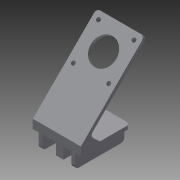
# Autodesk Inventor part: slider
Saved by Autodesk Inventor 2015 (Build 190159000, 159)
## iProperties
Created: 2014-11-15
Part Number: slider
Material: Generic
Document SubType Name: Modeling
Designer: Rene
Density: 1 g/cm^3
Appearance: Default
Author: Rene
Autodesk Inventor part; units mm, degrees
ref_plane "YZ Plane" through (0, 0, 0) normal (1, 0, 0) x (0, 1, 0)
ref_plane "XZ Plane" through (0, 0, 0) normal (0, 1, 0) x (-1, 0, 0)
ref_plane "XY Plane" through (0, 0, 0) normal (0, 0, 1) x (1, 0, 0)
sketch "Sketch1" plane through (0, 0, 0) normal (0, 1, 0) x (-1, 0, 0)
  line L0 (9.3294, -16.9333) -> (-32.5806, -16.9333)
  line L1 (-32.5806, -16.9333) -> (-32.5806, 33.8667)
  line L2 (-32.5806, 33.8667) -> (9.3294, 33.8667)
  line L3 (9.3294, 33.8667) -> (9.3294, -16.9333)
  point P0 (0, 0)
  dimension "d0" = 50.8
  dimension "d1" = 41.91
  constraints: 8 end point, 2 parallel, 1 horizontal, 1 perpendicular
  measures "d0" distance of L0.end L1.end
  measures "d1" distance of L1.end L2.end
extrude "Extrusion1" add sketch "Sketch1" along normal blind 3.175
chamfer "Chamfer1" distance 3.175 angle 45 1 edges at (11.6256, 3.175, 33.8667)
sketch "Sketch9" plane through (32.5806, 0, -16.9333) normal (1, 0, 0) x (0, 0, -1)
  line L0 (-47.625, 3.175) -> (0, 3.175) projected
  line L1 (-11.631, 34.6788) -> (-43.1349, 3.175) projected
  line L2 (-13.8761, 36.9239) -> (-11.631, 34.6788) projected
  line L3 (-34.9797, 11.3302) -> (-26.8245, 3.175)
  point P0 (-16.9333, 0)
  dimension "d15" = 33.02
  constraints: 2 end point, 2 point on line, 1 parallel
  measures "d15" distance between parallel lines of L2 L3
extrude "Extrusion4" add sketch "Sketch9" against normal blind 3.175
sketch "Sketch10" plane through (-9.3294, 0, -16.9333) normal (-1, 0, 0) x (0, 0, 1)
  line L0 (0, 3.175) -> (47.625, 3.175) projected
  line L1 (13.8761, 36.9239) -> (11.631, 34.6788) projected
  line L2 (43.1349, 3.175) -> (11.631, 34.6788) projected
  line L3 (34.9797, 11.3302) -> (26.8245, 3.175)
  point P0 (16.9333, 0)
  dimension "d18" = 33.02
  constraints: 2 end point, 2 point on line, 1 perpendicular
  measures "d18" distance between parallel lines of L1 L3
extrude "Extrusion5" add sketch "Sketch10" against normal blind 3.175
fillet "Fillet3" radius 3.175 2 edges at (-7.7419, 3.175, 9.8912) (30.9931, 3.175, 9.8912)
fillet "Fillet4" radius 3.175 2 edges at (-9.3294, 1.5875, -16.9333) (32.5806, 1.5875, -16.9333)
sketch "Sketch11" plane through (0, 0, 0) normal (0, -1, 0) x (1, 0, 0)
  line L0 (-9.3294, 26.2015) -> (32.5806, 26.2015) projected
  line L1 (-9.3294, 33.8667) -> (-9.3294, -13.7583) projected
  line L2 (-6.1544, -16.9333) -> (29.4056, -16.9333) projected
  line L3 (32.5806, -13.7583) -> (32.5806, 33.8667) projected
  line L4 (11.6256, 26.2015) -> (11.6256, -16.9333)
  line L5 (-9.3294, 0.8015) -> (32.5806, 0.8015)
  circle A0 centre (11.6256, 0.8015) radius 3.175
  point P0 (0, 0)
  dimension "d24" = 20.955
  dimension "d25" = 25.4
  dimension "d26" = 6.35
  constraints: 4 end point, 3 midpoint, 2 point on line, 1 centre point, 1 perpendicular
  measures "d24" distance between parallel lines of L1 L4
  measures "d25" distance between parallel lines of L0 L5
  measures "d26" diameter of A0
extrude "Extrusion9" cut sketch "Sketch11" against normal blind 12.446 contours A0 L5 L4 | L4 L5 A0 | L5 L4 A0 | L5 A0 L4
sketch "Sketch19" plane through (0, 0, 0) normal (0, -1, 0) x (1, 0, 0)
  circle A0 centre (11.6256, 0.8015) radius 3.175 projected
  circle A1 centre (11.6256, -9.3585) radius 3.175
  point P0 (0, 0)
  dimension "d44" = 6.35
  dimension "d45" = 10.16
  dimension "d46" = 0
  constraints: 1 centre point
  measures "d44" diameter of A1
  measures "d45" distance of A0.centre A1.centre
  measures "d46" horizontal distance of A0.centre A1.centre
extrude "Extrusion10" add sketch "Sketch19" along normal blind 12.446 contours A1
sketch "Sketch20" plane through (0, 0, 0) normal (0, -1, 0) x (1, 0, 0)
  circle A0 centre (11.6256, 0.8015) radius 3.175 projected
  circle A1 centre (11.6256, 10.9615) radius 3.175
  point P0 (0, 0)
  dimension "d49" = 6.35
  dimension "d50" = 10.16
  dimension "d51" = 0
  constraints: 1 centre point
  measures "d49" diameter of A1
  measures "d50" distance of A0.centre A1.centre
  measures "d51" horizontal distance of A0.centre A1.centre
extrude "Extrusion11" add sketch "Sketch20" along normal blind 12.446 contours A1
sketch "Sketch24" plane through (0, 0, 0) normal (0, -1, 0) x (1, 0, 0)
  circle A0 centre (11.6256, 0.8015) radius 3.175 projected
  line L0 (-9.3294, 26.2015) -> (32.5806, 26.2015) projected
  line L1 (-6.1544, -16.9333) -> (29.4056, -16.9333) projected
  line L2 (24.3256, 26.2015) -> (24.3256, -16.9333)
  line L3 (24.3256, 26.2015) -> (27.5006, 26.2015)
  line L4 (27.5006, 26.2015) -> (27.5006, -16.9333)
  line L5 (27.5006, -16.9333) -> (24.3256, -16.9333)
  line L6 (24.3256, -16.9333) -> (24.3256, 26.2015)
  point P0 (0, 0)
  dimension "d64" = 12.7
  dimension "d65" = 3.175
  constraints: 10 end point, 3 point on line, 2 parallel, 2 perpendicular, 1 horizontal
  measures "d64" distance from line of L2 A0.centre
  measures "d65" distance of L2.start L3.end
extrude "Extrusion14" add sketch "Sketch24" along normal blind 12.446 contours L0 L4 L1 L2
sketch "Sketch25" plane through (0, 0, 0) normal (0, -1, 0) x (1, 0, 0)
  circle A0 centre (11.6256, 0.8015) radius 3.175 projected
  line L0 (-9.3294, 26.2015) -> (24.3256, 26.2015) projected
  line L1 (-6.1544, -16.9333) -> (24.3256, -16.9333) projected
  line L2 (-1.0744, 26.2015) -> (-1.0744, -16.9333)
  line L3 (-1.0744, -16.9333) -> (-4.2494, -16.9333)
  line L4 (-4.2494, -16.9333) -> (-4.2494, 26.2015)
  line L5 (-4.2494, 26.2015) -> (-1.0744, 26.2015)
  line L6 (-1.0744, 26.2015) -> (-1.0744, -16.9333)
  point P0 (0, 0)
  dimension "d68" = 12.7
  dimension "d69" = 3.175
  constraints: 10 end point, 3 point on line, 2 parallel, 2 perpendicular, 1 horizontal
  measures "d68" distance from line of L2 A0.centre
  measures "d69" distance between parallel lines of L6 L4
extrude "Extrusion15" add sketch "Sketch25" along normal blind 12.446 contours L0 L2 L1 L4
fillet "Fillet8" radius 3.175 4 edges at (25.9131, -12.446, 26.2015) (25.9131, -12.446, -16.9333) (-2.6619, -12.446, -16.9333) (-2.6619, -12.446, 26.2015)
sketch "Sketch28" plane through (-9.3294, 3.175, 30.6917) normal (0, 0.7071068, 0.7071068) x (1, 0, 0)
  line L0 (41.91, -4.4901) -> (41.91, 0) projected
  line L1 (41.91, 0) -> (0, 0) projected
  line L2 (0, 0) -> (0, -4.4901) projected
  line L3 (41.91, -4.4901) -> (0, -4.4901) projected
  line L4 (0, -4.4901) -> (41.91, -4.4901)
  line L5 (41.91, -4.4901) -> (41.91, 85.0449)
  line L6 (41.91, 85.0449) -> (0, 85.0449)
  line L7 (0, 85.0449) -> (0, -4.4901)
  point P0 (9.3294, 19.4572)
  dimension "d75" = 41.91
  dimension "d76" = 89.535
  constraints: 8 end point, 2 parallel, 1 horizontal, 1 perpendicular
  measures "d75" distance between parallel lines of L5 L7
  measures "d76" distance between parallel lines of L3 L6
extrude "Extrusion16" add sketch "Sketch28" against normal blind 3.175 contours L1 L7 L6 L5
sketch "Sketch29" plane through (-9.3294, 0, 33.8667) normal (0, 0.7071068, 0.7071068) x (1, 0, 0)
  line L0 (41.91, 89.535) -> (0, 89.535) projected
  line L1 (0, 89.535) -> (0, 0) projected
  circle A0 centre (20.955, 68.58) radius 11.1125
  point P0 (9.3294, 23.9473)
  dimension "d79" = 22.225
  dimension "d80" = 20.955
  dimension "d81" = 20.955
  constraints: 1 centre point
  measures "d79" diameter of A0
  measures "d80" distance from line of L1 A0.centre
  measures "d81" distance from line of L0 A0.centre
extrude "Extrusion17" cut sketch "Sketch29" against normal blind 3.175
sketch "Sketch30" plane through (-9.3294, 0, 33.8667) normal (0, 0.7071068, 0.7071068) x (1, 0, 0)
  circle A0 centre (20.955, 68.58) radius 11.1125 projected
  circle A1 centre (5.461, 84.074) radius 1.7272
  point P0 (9.3294, 23.9473)
  dimension "d84" = 3.4544
  dimension "d85" = 15.494
  dimension "d86" = 15.494
  constraints: 1 centre point
  measures "d84" diameter of A1
  measures "d85" horizontal distance of A0.centre A1.centre
  measures "d86" horizontal distance of A0.centre A1.centre
extrude "Extrusion18" cut sketch "Sketch30" against normal blind 3.175 contours A1
sketch "Sketch31" plane through (-9.3294, 0, 33.8667) normal (0, 0.7071068, 0.7071068) x (1, 0, 0)
  circle A0 centre (5.461, 84.074) radius 1.7272 projected
  circle A1 centre (20.955, 68.58) radius 11.1125 projected
  circle A2 centre (5.461, 53.086) radius 1.7272
  point P0 (9.3294, 23.9473)
  dimension "d89" = 3.4544
  dimension "d90" = 3.4544
  dimension "d91" = 15.494
  dimension "d92" = 15.494
  constraints: 1 centre point
  measures "d89" diameter of A0
  measures "d90" diameter of A2
  measures "d91" horizontal distance of A1.centre A2.centre
  measures "d92" horizontal distance of A1.centre A2.centre
extrude "Extrusion19" cut sketch "Sketch31" against normal blind 3.175 contours A2
sketch "Sketch32" plane through (-9.3294, 0, 33.8667) normal (0, 0.7071068, 0.7071068) x (1, 0, 0)
  circle A0 centre (20.955, 68.58) radius 11.1125 projected
  circle A1 centre (36.449, 84.074) radius 1.7272
  point P0 (9.3294, 23.9473)
  dimension "d95" = 3.4544
  dimension "d96" = 15.494
  dimension "d97" = 15.494
  constraints: 1 centre point
  measures "d95" diameter of A1
  measures "d96" horizontal distance of A1.centre A0.centre
  measures "d97" horizontal distance of A0.centre A1.centre
extrude "Extrusion20" cut sketch "Sketch32" against normal blind 3.175 contours A1
sketch "Sketch33" plane through (-9.3294, 0, 33.8667) normal (0, 0.7071068, 0.7071068) x (1, 0, 0)
  circle A0 centre (20.955, 68.58) radius 11.1125 projected
  circle A1 centre (36.449, 53.086) radius 1.7272
  point P0 (9.3294, 23.9473)
  dimension "d100" = 3.4544
  dimension "d101" = 15.494
  dimension "d102" = 15.494
  constraints: 1 centre point
  measures "d100" diameter of A1
  measures "d101" horizontal distance of A1.centre A0.centre
  measures "d102" horizontal distance of A0.centre A1.centre
extrude "Extrusion21" cut sketch "Sketch33" against normal blind 3.175 contours A1
fillet "Fillet9" radius 3.175 2 edges at (-9.3294, 62.1883, -30.5667) (32.5806, 62.1883, -30.5667)
fillet "Fillet10" radius 3.175 2 edges at (30.9931, 11.3302, 18.0464) (-7.7419, 11.3302, 18.0464)
sketch "Sketch37" plane through (11.6256, -12.446, 10.9615) normal (0, -1, 0) x (1, 0, 0)
  line L0 (-15.875, 12.065) -> (-15.875, -24.7199) projected
  line L1 (-12.7, -24.7199) -> (-12.7, 12.065) projected
  circle A0 centre (0, 0) radius 3.175 projected
  line L2 (-3.175, 0) -> (3.175, 0)
  line L3 (3.175, 0) -> (3.175, 12.7)
  line L4 (3.175, 12.7) -> (-3.175, 12.7)
  line L5 (-3.175, 12.7) -> (-3.175, 0)
  point P0 (-11.6256, -10.9615)
  dimension "d111" = 3.175
  dimension "d112" = 6.35
  dimension "d113" = 12.7
  constraints: 8 end point, 2 parallel, 1 horizontal, 1 horizontal alignment, 1 perpendicular, 1 other
  measures "d111" distance between parallel lines of L0 L1
  measures "d112" distance between parallel lines of L5 L3
  measures "d113" distance of L4.end L2.start
extrude "Extrusion22" add sketch "Sketch37" against normal blind 12.954 contours L2 A0 | A0 L5 L4 L3 picked at (0.7922, 0.7018)
sketch "Sketch38" plane through (0, -12.446, 0) normal (0, -1, 0) x (1, 0, 0)
  line L0 (14.8006, 10.9615) -> (14.8006, 23.6615) projected
  line L1 (14.8006, 16.2386) -> (8.4506, 16.2386)
  line L2 (8.4506, 16.2386) -> (8.4506, 7.2793)
  line L3 (8.4506, 7.2793) -> (14.8006, 7.2793)
  line L4 (14.8006, 7.2793) -> (14.8006, 16.2386)
  point P0 (0, 0)
  dimension "d116" = 6.35
  constraints: 8 end point, 2 parallel, 1 horizontal, 1 perpendicular, 1 point on line
  measures "d116" distance between parallel lines of L2 L0
extrude "Extrusion23" add sketch "Sketch38" against normal blind 12.954
sketch "Sketch39" plane through (11.6256, -12.446, -9.3585) normal (0, -1, 0) x (1, 0, 0)
  line L0 (3.175, -3.175) -> (-3.175, -3.175)
  line L1 (-3.175, -3.175) -> (-3.175, 3.175)
  line L2 (-3.175, 3.175) -> (3.175, 3.175)
  line L3 (3.175, 3.175) -> (3.175, -3.175)
  point P0 (-11.6256, 9.3585)
  dimension "d119" = 6.35
  dimension "d120" = 6.35
  constraints: 8 end point, 2 parallel, 1 horizontal, 1 perpendicular
  measures "d119" distance of L0.end L1.end
  measures "d120" distance between parallel lines of L1 L3
extrude "Extrusion24" add sketch "Sketch39" against normal blind 12.954
fillet "Fillet12" radius 3.175 1 edges at (14.8006, -6.223, -12.5335)
fillet "Fillet13" radius 3.175 1 edges at (8.4506, -6.223, -12.5335)
sketch "Sketch44" plane through (32.5806, 0, 33.8667) normal (1, 0, 0) x (0, 0, -1)
  line L0 (7.6651, 0) -> (7.6651, 7.6651)
  line L1 (61.0657, 61.0657) -> (0, 0) projected
  line L2 (0, 0) -> (7.6651, 0)
  line L3 (47.625, 0) -> (0, 0) projected
  line L4 (7.6651, 7.6651) -> (0, 0)
  point P0 (33.8667, 0)
  constraints: 6 end point, 2 collinear, 1 point on line, 1 vertical
extrude "Extrusion25" cut sketch "Sketch44" against normal blind 76.2
sketch "Sketch45" plane through (-9.3294, 0.9299, 28.4466) normal (0, -0.7071068, -0.7071068) x (-1, 0, 0)
  line L0 (-38.735, 3.175) -> (-3.175, 3.175)
  line L1 (-3.175, 3.175) -> (-3.175, 34.1687)
  line L2 (-3.175, 34.1687) -> (-38.735, 34.1687)
  line L3 (-38.735, 34.1687) -> (-38.735, 3.175)
  line L4 (-3.175, 3.175) -> (-3.175, 17.8832) projected
  circle A0 centre (-36.449, 48.5959) radius 1.7272 projected
  point P0 (-9.3294, 19.4572)
  dimension "d129" = 0
  dimension "d130" = 12.7
  constraints: 8 end point, 2 parallel, 1 horizontal, 1 perpendicular
  measures "d129" distance between parallel lines of L4 L1
  measures "d130" distance edge to line of A0 L2
extrude "Extrusion26" add sketch "Sketch45" along normal blind 3.81 contours L3 L2 L1 L0
chamfer "Chamfer2" distance 3.81 angle 45 1 edges at (11.6256, 22.3968, 1.5916)
fillet "Fillet14" radius 3.175 1 edges at (11.6256, 3.175, 20.8134)
sketch "Sketch47" plane through (0, -12.446, 0) normal (0, -1, 0) x (1, 0, 0)
  line L0 (14.8006, -6.1835) -> (8.4506, -6.1835)
  line L1 (8.4506, -6.1835) -> (8.4506, -12.6132)
  line L2 (8.4506, -12.6132) -> (14.8006, -12.6132)
  line L3 (14.8006, -12.6132) -> (14.8006, -6.1835)
  point P0 (0, 0)
  constraints: 8 end point, 2 parallel, 1 horizontal, 1 perpendicular
extrude "Extrusion27" cut sketch "Sketch47" against normal blind 12.446
body "Solid1"
